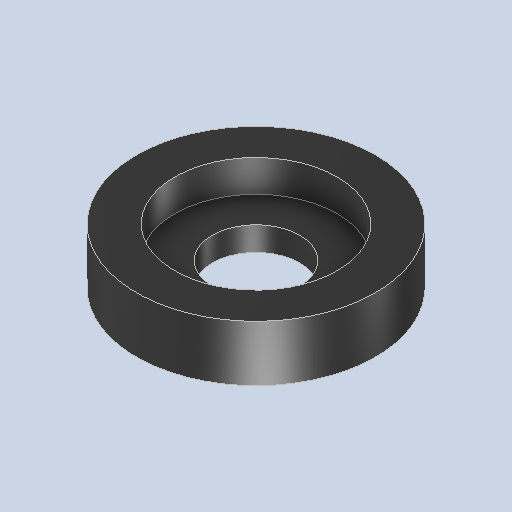
# Autodesk Inventor part: UZB
Saved by Autodesk Inventor 2024.2 (Build 282272000, 272)
## iProperties
Created: 2024-01-05
Part Number: UZB
Material: Stainless Steel
Document SubType Name: Modeling
Designer: Masato Kubotera
Density: 8 g/cm^3
Appearance: Glossy - Black
Catalog Web Link: https://jp.misumi-ec.com/vona2/detail/110300521530/?ProductCode=UZB
Vendor: MISUMI
Mass: 3.3555 g
Surface Area: 5.60853 cm^2
Volume: 0.419438 cm^3
Author: Masato Kubotera
Autodesk Inventor part; units mm, degrees
ref_plane "YZ Plane" through (0, 0, 0) normal (1, 0, 0) x (0, 1, 0)
ref_plane "XZ Plane" through (0, 0, 0) normal (0, 1, 0) x (-1, 0, 0)
ref_plane "XY Plane" through (0, 0, 0) normal (0, 0, 1) x (1, 0, 0)
sketch "Sketch1" plane through (0, 0, 0) normal (0, 1, 0) x (-1, 0, 0)
  line L0 (0, 0) -> (0, 3.5)
  line L1 (5.1, 3.5) -> (7.5, 3.5)
  line L2 (7.5, 3.5) -> (7.5, 0)
  line L3 (7.5, 0) -> (2.75, 0)
  line L4 (2.75, 1.5) -> (5.1, 1.5)
  line L5 (5.1, 1.5) -> (5.1, 3.5)
  line L6 (2.75, 1.5) -> (2.75, 0)
  dimension "d0" = 15
  dimension "d1" = 10.2
  dimension "d2" = 5.5
  dimension "d3" = 2
  dimension "d4" = 3.5
  constraints: 14 end point, 4 vertical, 3 horizontal, 2 point on line
  measures "d0" diameter of L2 L0
  measures "d1" diameter of L5 L0
  measures "d2" diameter of L6 L0
  measures "d3" distance of L4.end L1.start
  measures "d4" distance of L1.end L2.end
revolve "Revolution1" add sketch "Sketch1" angle 360 about axis through (0, 0, 0) along (0, 0, 1)
body "Solid1"
